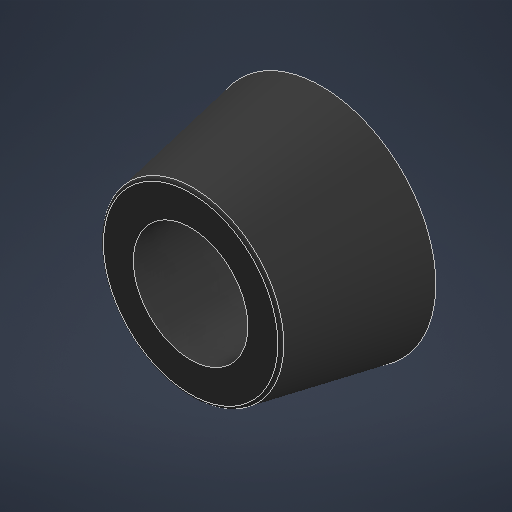
# Autodesk Inventor part: Amortecedor_Borracha
Saved by Autodesk Inventor 2025.2 (Build 292293000, 293)
## iProperties
Created: 2025-05-14
Part Number: Amortecedor_Borracha
Material: Rubber
Document SubType Name: Modeling
Designer: Tiago
Density: 0.93 g/cm^3
Appearance: Rubber - Black
Mass: 0.316559 g
Surface Area: 5.88279 cm^2
Volume: 0.340386 cm^3
Author: Tiago
Autodesk Inventor part; units mm, degrees
ref_plane "YZ Plane" through (0, 0, 0) normal (1, 0, 0) x (0, 1, 0)
ref_plane "XZ Plane" through (0, 0, 0) normal (0, 1, 0) x (-1, 0, 0)
ref_plane "XY Plane" through (0, 0, 0) normal (0, 0, 1) x (1, 0, 0)
sketch "Sketch1" plane through (0, 0, 0) normal (0, 0, 1) x (1, 0, 0)
  circle A0 centre (0, 0) radius 3.5
  circle A1 centre (0, 0) radius 1.5
  circle A2 centre (0, 0) radius 3.05
  dimension "D" = 7
  dimension "M3" = 3
  dimension "d12" = 6.1
  constraints: 3 centre point, 3 coincident
  measures "D" diameter of A0
  measures "M3" diameter of A1
  measures "d12" diameter of A2
extrude "Extrusion1" add sketch "Sketch1" along normal blind 8 contours A0 | A2
sketch "Sketch3" plane through (0, 0, 0) normal (1, 0, 0) x (0, 1, 0)
  line L0 (3.5, 8) -> (3.5, 0) projected
  line L1 (3.5, 0) -> (1.5, 0) projected
  line L2 (1.5, 0) -> (1.5, 8) projected
  line L3 (1.5, 8) -> (3.5, 8) projected
  line L4 (-3.5, 0) -> (-3.5, 8) projected
  line L5 (-3.5, 8) -> (-1.5, 8) projected
  line L6 (-1.5, 8) -> (-1.5, 0) projected
  line L7 (-1.5, 0) -> (-3.5, 0) projected
  line L8 (5.6436, 0) -> (3.5, 0)
  line L9 (0, -1.6) -> (0, 9.6) projected
  line L10 (3.5, 8) -> (5.5, 8)
  line L11 (5.5, 8) -> (7, 0)
  line L12 (7, 0) -> (3.5, 0)
  point P0 (0, 0)
  dimension "d15" = 2
  dimension "d18" = 7
  constraints: 8 end point, 1 collinear, 1 horizontal, 1 perpendicular
  measures "d15" distance of L0.start L10.end
  measures "d18" distance of point (0, 0) L11.end
revolve "Revolution2" add sketch "Sketch3" angle 360 about axis through (0, 0, -10) along (0, 0, 1) contours L10 L11 L12 L8 L0
extrude "Extrusion3" cut sketch "Sketch1" along normal up to surface (8 mm away) contours A0 | A2
fillet "Fillet1" radius 0.2 1 edges at (0, -5.5, 8)
extrude "Extrusion4" add sketch "Sketch1" along normal blind 1.5 contours A0 | A2
body "Solid1"
